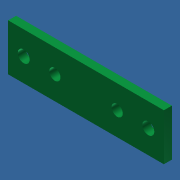
# Autodesk Inventor part: J002609
Saved by Autodesk Inventor 2012 SP2 (Build 160219200, 219)
## iProperties
Created: 2014-07-01
Material: Default
Vendor: HHMI: JFRC - ID&F
Document SubType Name: Modeling
Designer: NEGRASHOVI
Density: 1 g/cm^3
Part Number: J002609
RuleStatus: InUse
AfterDocSave0: file://Part Number Cleaner
DESIGN DEPARTMENT: HHMI: JFRC - ID&F
ALTERED ITEM PART NUMBER: N/A
ALTERED ITEM VENDOR: N/A
ALTERED ITEM DESCRIPTION: N/A
Author: NEGRASHOVI
Revision Number: 0
Autodesk Inventor part; units mm, degrees
ref_plane "YZ Plane" through (0, 0, 0) normal (1, 0, 0) x (0, 1, 0)
ref_plane "XZ Plane" through (0, 0, 0) normal (0, 1, 0) x (-1, 0, 0)
ref_plane "XY Plane" through (0, 0, 0) normal (0, 0, 1) x (1, 0, 0)
sketch "Sketch1" plane through (0, 0, 0) normal (0, 0, 1) x (1, 0, 0)
  line L0 (-15.875, -4.7625) -> (15.875, -4.7625)
  line L1 (15.875, -4.7625) -> (15.875, 4.7625)
  line L2 (15.875, 4.7625) -> (-15.875, 4.7625)
  line L3 (-15.875, 4.7625) -> (-15.875, -4.7625)
  line L4 (-15.875, -4.7625) -> (15.875, 4.7625) construction
  point P0 (0, 0)
  point P1 (0, 0)
  dimension "d0" = 9.525
  dimension "d1" = 31.75
  constraints: 10 end point, 2 parallel, 1 coincident, 1 horizontal, 1 midpoint, 1 perpendicular
  measures "d0" distance of L2.end L0.start
  measures "d1" distance of L1.end L2.end
extrude "Extrusion1" add sketch "Sketch1" along normal blind 1.6256
sketch "Sketch2" plane through (0, 0, 1.6256) normal (0, 0, 1) x (1, 0, 0)
  line L0 (-22.225, 0) -> (22.225, 0) construction
  line L1 (0, -6.6675) -> (0, 6.6675) construction
  point P0 (0, 0)
  point P1 (-12.7, 0)
  point P2 (12.7, 0)
  dimension "d4" = 25.4
  constraints: 2 point on line, 1 symmetric about line
  measures "d4" distance of point (12.7, 0) point (-12.7, 0)
hole "Hole1" at (-12.7, 0, 1.6256) at (12.7, 0, 1.6256) direction (0, 0, -1) diameter 2.4384 end through all clearance for "Flat Head Machine Screw (82)" size "#2" standard "Ansi Unified Screw Threads"
sketch "Sketch3" plane through (0, 0, 1.6256) normal (0, 0, 1) x (1, 0, 0)
  line L0 (-22.225, 0) -> (22.225, 0) construction
  line L1 (0, -6.6675) -> (0, 6.6675) construction
  point P0 (0, 0)
  point P1 (-6.35, 0)
  point P2 (6.35, 0)
  dimension "d12" = 12.7
  constraints: 2 point on line, 1 symmetric about line
  measures "d12" distance of point (-6.35, 0) point (6.35, 0)
hole "Hole2" at (-6.35, 0, 1.6256) at (6.35, 0, 1.6256) direction (0, 0, -1) diameter 2.286 end through all
body "Solid1"
